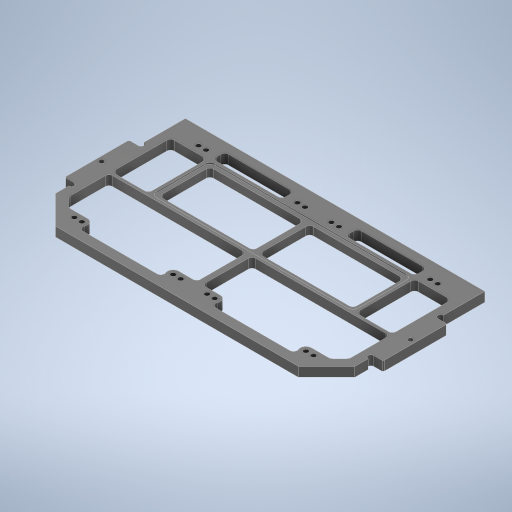
# Autodesk Inventor part: TorsoElectronicBoxBoardMountFrame
Saved by Autodesk Inventor 2024.2 (Build 282272000, 272)
## iProperties
Created: 2024-01-11
Part Number: TorsoElectronicBoxBoardMountFrame
Material: Acetal Resin, Black
Document SubType Name: Modeling
Designer: Masato Kubotera
Density: 1.425 g/cm^3
Appearance: Smooth - Black
Vendor: meviy
Mass: 32.4012 g
Surface Area: 177.402 cm^2
Volume: 22.7377 cm^3
Author: Masato Kubotera
Autodesk Inventor part; units mm, degrees
ref_plane "YZ Plane" through (0, 0, 0) normal (1, 0, 0) x (0, 1, 0)
ref_plane "XZ Plane" through (0, 0, 0) normal (0, 1, 0) x (-1, 0, 0)
ref_plane "XY Plane" through (0, 0, 0) normal (0, 0, 1) x (1, 0, 0)
sketch "Sketch1" plane through (0, 0, 0) normal (0, 0, 1) x (1, 0, 0)
  line L0 (-42, -79.5) -> (42, -79.5)
  line L1 (42, -79.5) -> (42, 79.5)
  line L2 (42, 79.5) -> (-42, 79.5) construction
  line L3 (-42, 79.5) -> (-42, -79.5)
  line L4 (-42, -79.5) -> (42, 79.5) construction
  line L5 (42, -79.5) -> (-42, 79.5) construction
  line L6 (-42, 0) -> (42, 0)
  line L7 (-17, 84.5) -> (17, 84.5)
  line L8 (17, 84.5) -> (17, 79.5)
  line L9 (-17, 84.5) -> (-17, 79.5)
  arc A0 (-20, 79.5) -> (-17, 79.5) centre (-18.5, 79.5) ccw
  line L10 (17, 84.5) -> (17, 79.5)
  arc A1 (17, 79.5) -> (20, 79.5) centre (18.5, 79.5) ccw
  line L11 (0, 79.5) -> (0, 84.5) construction
  line L12 (0, -70) -> (0, 70) construction
  line L13 (-33, 7) -> (33, 7) construction
  line L14 (33, 7) -> (33, 63.5) construction
  line L15 (33, 63.5) -> (-33, 63.5) construction
  line L16 (-33, 63.5) -> (-33, 7) construction
  line L17 (-33, 7) -> (33, 63.5) construction
  line L18 (33, 7) -> (-33, 63.5) construction
  line L19 (-40, 2.75) -> (40, 2.75) construction
  line L20 (40, 2.75) -> (40, 67.75) construction
  line L21 (40, 67.75) -> (-40, 67.75) construction
  line L22 (-40, 67.75) -> (-40, 2.75) construction
  line L23 (-40, 2.75) -> (40, 67.75) construction
  line L24 (40, 2.75) -> (-40, 67.75) construction
  line L25 (-40, 35.25) -> (40, 35.25) construction
  line L26 (5.6, 74.5) -> (24.1005, 74.5)
  line L27 (30, 11) -> (30, 3.5)
  arc A2 (34.2, 13.7495) -> (37, 15.5826) centre (35, 15.5826) ccw
  arc A3 (28, 1.5) -> (30, 3.5) centre (28, 3.5) ccw
  line L28 (-42, 79.5) -> (-20, 79.5)
  line L29 (20, 79.5) -> (42, 79.5)
  line L30 (-26, -53.5) -> (-1, -53.5) construction
  line L31 (2, -50.5) -> (2, 50.5) construction
  line L32 (-1, 53.5) -> (-26, 53.5) construction
  line L33 (-29, 50.5) -> (-29, -50.5) construction
  arc A4 (-26, 53.5) -> (-29, 50.5) centre (-26, 50.5) ccw construction
  arc A5 (2, 50.5) -> (-1, 53.5) centre (-1, 50.5) ccw construction
  arc A6 (-29, -50.5) -> (-26, -53.5) centre (-26, -50.5) ccw construction
  arc A7 (-1, -53.5) -> (2, -50.5) centre (-1, -50.5) ccw construction
  line L34 (-29, 0) -> (2, 0) construction
  circle A8 centre (-33, 7) radius 3 construction
  line L35 (-13.5, 53.5) -> (-13.5, -53.5) construction
  line L36 (5.6, 1.5) -> (28, 1.5)
  arc A9 (5.6, 74.5) -> (3.6, 72.5) centre (5.6, 72.5) ccw
  line L37 (-25, 1.5) -> (-2, 1.5)
  line L38 (0, 3.5) -> (0, 49.5)
  line L39 (-2, 51.5) -> (-25, 51.5)
  line L40 (-27, 49.5) -> (-27, 3.5)
  arc A10 (-27, 3.5) -> (-25, 1.5) centre (-25, 3.5) ccw
  arc A11 (-2, 1.5) -> (0, 3.5) centre (-2, 3.5) ccw
  arc A12 (0, 49.5) -> (-2, 51.5) centre (-2, 49.5) ccw
  arc A13 (-25, 51.5) -> (-27, 49.5) centre (-25, 49.5) ccw
  line L41 (30, 59.5) -> (30, 68.6005)
  arc A14 (30, 59.5) -> (34.2, 56.7505) centre (33, 59.5) ccw
  arc A15 (37, 54.9174) -> (34.2, 56.7505) centre (35, 54.9174) ccw
  line L42 (37, 54.9174) -> (37, 15.5826)
  arc A16 (34.2, 13.7495) -> (30, 11) centre (33, 11) ccw
  line L43 (-29.1, 0) -> (-29.1, 50.6)
  line L44 (-26.1, 53.6) -> (-0.9, 53.6)
  line L45 (2.1, 50.6) -> (2.1, 0)
  arc A17 (2.1, 50.6) -> (-0.9, 53.6) centre (-0.9, 50.6) ccw
  arc A18 (-26.1, 53.6) -> (-29.1, 50.6) centre (-26.1, 50.6) ccw
  line L46 (3.6, 3.5) -> (3.6, 72.5)
  arc A19 (3.6, 3.5) -> (5.6, 1.5) centre (5.6, 3.5) ccw
  line L47 (-27.1, 55.1) -> (0.1, 55.1)
  line L48 (2.1, 57.1) -> (2.1, 72.5)
  line L49 (0.1, 74.5) -> (-27.1, 74.5)
  line L50 (-29.1, 72.5) -> (-29.1, 57.1)
  line L51 (-35, 16.9) -> (-32.6, 16.9)
  line L52 (-30.6, 18.9) -> (-30.6, 51.6)
  line L53 (-32.6, 53.6) -> (-35, 53.6)
  line L54 (-37, 51.6) -> (-37, 18.9)
  circle A20 centre (-33, 11) radius 3 construction
  circle A21 centre (-33, 59.5) radius 3 construction
  arc A22 (-29.1, 57.1) -> (-27.1, 55.1) centre (-27.1, 57.1) ccw
  arc A23 (0.1, 55.1) -> (2.1, 57.1) centre (0.1, 57.1) ccw
  arc A24 (2.1, 72.5) -> (0.1, 74.5) centre (0.1, 72.5) ccw
  arc A25 (-27.1, 74.5) -> (-29.1, 72.5) centre (-27.1, 72.5) ccw
  arc A26 (-30.6, 51.6) -> (-32.6, 53.6) centre (-32.6, 51.6) ccw
  arc A27 (-35, 53.6) -> (-37, 51.6) centre (-35, 51.6) ccw
  arc A28 (-37, 18.9) -> (-35, 16.9) centre (-35, 18.9) ccw
  arc A29 (-32.6, 16.9) -> (-30.6, 18.9) centre (-32.6, 18.9) ccw
  line L55 (27, 79.5) -> (42, 64.5)
  line L56 (29.4142, 70.0147) -> (25.5147, 73.9142)
  arc A30 (30, 68.6005) -> (29.4142, 70.0147) centre (28, 68.6005) ccw
  arc A31 (25.5147, 73.9142) -> (24.1005, 74.5) centre (24.1005, 72.5) ccw
  point P0 (0, 0)
  point P1 (0, 35.25)
  point P2 (0, 82)
  point P3 (-29, -53.5)
  point P4 (2, -53.5)
  point P5 (-29.1, 55.1)
  point P6 (2.1, 74.5)
  point P7 (2.1, 55.1)
  point P8 (-29.1, 74.5)
  point P9 (-37, 16.9)
  point P10 (-30.6, 53.6)
  point P11 (-30.6, 16.9)
  point P12 (-37, 53.6)
  dimension "d1" = 159
  dimension "d2" = 1.5
  dimension "d3" = 5
  dimension "d36" = 25
  dimension "d42" = 56.5
  dimension "d43" = 66
  dimension "d44" = 80
  dimension "d45" = 65
  dimension "d67" = 5
  dimension "d70" = 42
  dimension "d71" = 84
  dimension "d73" = 25
  dimension "d75" = 14
  dimension "d95" = 3
  dimension "d97" = 31
  dimension "d100" = 107
  dimension "d102" = 6
  dimension "d103" = 1
  dimension "d108" = 3
  dimension "d113" = 2
  dimension "d114" = 2
  dimension "d115" = 2
  dimension "d116" = 5
  dimension "d117" = 4
  dimension "d118" = 6
  dimension "d122" = 2
  dimension "d123" = 0.1
  dimension "d124" = 0.1
  dimension "d131" = 1.5
  dimension "d143" = 1.5
  dimension "d147" = 15
  dimension "d148" = 45
  dimension "d150" = 5
  constraints: 114 end point, 58 point on circle, 49 tangent, 32 centre point, 31 point on line, 23 equal radius, 18 midpoint, 13 parallel, 12 horizontal, 10 vertical, 9 coincident, 8 collinear, 7 symmetric about line, 6 perpendicular, 8 other
  measures "d1" distance of L1.end L0.end
  measures "d2" radius of A0
  measures "d3" distance of L7.start L9.end
  measures "d36" distance between parallel lines of L8 L1
  measures "d42" distance of L15.end L13.start
  measures "d43" distance of L14.end L15.end
  measures "d44" distance of L21.end L20.end
  measures "d45" distance of L19.end L20.end
  measures "d67" distance between parallel lines of L2 L26
  measures "d70" distance between parallel lines of L1 L12
  measures "d71" distance between parallel lines of L1 L3
  measures "d73" distance between parallel lines of L9 L3
  measures "d75" diameter of point (-33, 7) L6
  measures "d95" radius of A4
  measures "d97" distance of point (-29, -53.5) point (2, -53.5)
  measures "d100" distance between parallel lines of L32 L30
  measures "d102" diameter of A8
  measures "d103" distance edge to line of A8 L33
  measures "d108" diameter of L36 L6
  measures "d113" radius of A10
  measures "d114" distance between parallel lines of L31 L38
  measures "d115" distance between parallel lines of L32 L39
  measures "d116" distance between parallel lines of L1 L42
  measures "d117" distance of point (33, 11) point (33, 7)
  measures "d118" diameter of A16
  measures "d122" radius of A3
  measures "d123" distance between parallel lines of L45 L31
  measures "d124" distance between parallel lines of L44 L32
  measures "d131" distance between parallel lines of L46 L45
  measures "d143" distance between parallel lines of L47 L44
  measures "d147" distance of L1.end L55.end
  measures "d148" angle of L1 L55
  measures "d150" distance between parallel lines of L55 L56
extrude "Extrusion1" add sketch "Sketch1" against normal blind 5 contours L3 L28 A0 L9 L7 L8 A1 L29 L55 L1 L6 L45 A17 L44 A18 L43 | L43 A18 L44 A17 L45 L6
extrude "Extrusion2" cut sketch "Sketch1" against normal blind 0.7 contours L43 A18 L44 A17 L45 L6
chamfer "C0.5" distance 0.5 angle 45 2 edges at (17, 84.5, -2.5) (-17, 84.5, -2.5)
hole "M3" at (-33, 7, 0) at (-33, 63.5, 0) at (33, 7, 0) at (33, 63.5, 0) at (33, 11, 0) at (33, 59.5, 0) at (-33, 11, 0) at (-33, 59.5, 0) direction (0, 0, -1) diameter 2.459 end through all thread size "M3x0.5" class "6H" standard "ANSI Metric M Profile"
hole "Phi2.5" at (0, 82, 0) direction (0, 0, -1) diameter 2.5 end through all
mirror "Mirror1" about plane through (0, 0, 0) normal (0, 1, 0)
ref_plane "Work Plane1" through (-13.5, 53.5, 0) normal (-1, 0, 0) x (0, 0, 1)
body "Solid1"
